bruh_decora_1_v1 (Autodesk Fusion 360 design; units mm, degrees)
Autodesk Fusion 360 part; units mm, degrees
sketch "Sketch1" plane through (0, 0, 0) normal (0, 0, 1) x (1, 0, 0)
  line L0 (0, 0) -> (125, 0)
  line L1 (125, 0) -> (125, 123.4)
  line L2 (125, 123.4) -> (0, 123.4)
  line L3 (0, 123.4) -> (0, 0)
  line L4 (24.9, 95.1) -> (54.1, 95.1)
  line L5 (56.1, 93.1) -> (56.1, 30.3)
  line L6 (54.1, 28.3) -> (24.9, 28.3)
  line L7 (22.9, 30.3) -> (22.9, 93.1)
  line L8 (22.9, 61.7) -> (57.9534, 61.7)
  line L9 (56.1, 61.7) -> (57.9534, 61.7)
  circle A0 centre (39.5, 13.3) radius 3.5
  circle A1 centre (39.5, 110.1) radius 3.5
  circle A2 centre (39.5, 110.1) radius 1.5
  circle A3 centre (39.5, 13.3) radius 1.5
  line L10 (125, 61.7) -> (0, 61.7)
  arc A4 (22.9, 30.3) -> (24.9, 28.3) centre (24.9, 30.3) ccw
  arc A5 (54.1, 28.3) -> (56.1, 30.3) centre (54.1, 30.3) ccw
  arc A6 (56.1, 93.1) -> (54.1, 95.1) centre (54.1, 93.1) ccw
  arc A7 (24.9, 95.1) -> (22.9, 93.1) centre (24.9, 93.1) ccw
  line L11 (39.5, 123.4) -> (39.5, 0)
  circle A8 centre (85.5, 110.1) radius 1.5
  circle A9 centre (85.5, 110.1) radius 3.5
  circle A10 centre (85.5, 13.3) radius 3.5
  circle A11 centre (85.5, 13.3) radius 1.5
  line L12 (70.9, 28.3) -> (100.1, 28.3)
  line L13 (102.1, 30.3) -> (102.1, 93.1)
  line L14 (100.1, 95.1) -> (70.9, 95.1)
  line L15 (68.9, 93.1) -> (68.9, 30.3)
  line L16 (85.5, 123.4) -> (85.5, 0)
  line L17 (62.5, 0) -> (62.5, 123.4)
  arc A12 (102.1, 93.1) -> (100.1, 95.1) centre (100.1, 93.1) ccw
  arc A13 (70.9, 95.1) -> (68.9, 93.1) centre (70.9, 93.1) ccw
  arc A14 (100.1, 28.3) -> (102.1, 30.3) centre (100.1, 30.3) ccw
  arc A15 (68.9, 30.3) -> (70.9, 28.3) centre (70.9, 30.3) ccw
  point P0 (56.1, 95.1)
  point P1 (56.1, 28.3)
  point P2 (22.9, 28.3)
  point P3 (39.5, 28.3)
  point P4 (39.5, 95.1)
  point P5 (68.9, 28.3)
  point P6 (102.1, 28.3)
  point P7 (102.1, 95.1)
  point P8 (68.9, 61.7)
  point P9 (102.1, 61.7)
  point P10 (85.5, 95.1)
  point P11 (85.5, 28.3)
  dimension "d1" = 123.4
  dimension "d2" = 125
  dimension "d3" = 48.4
  dimension "d4" = 48.4
  dimension "d5" = 7
  dimension "d6" = 7
  dimension "d7" = 3
  dimension "d8" = 3
  dimension "d9" = 33.2
  dimension "d10" = 66.8
  dimension "d31" = 2
  dimension "d32" = 2
  dimension "d33" = 2
  dimension "d34" = 2
  dimension "d35" = 7
  dimension "d36" = 7
  dimension "d37" = 3
  dimension "d38" = 3
  dimension "d43" = 33.2
  dimension "d44" = 66.8
  dimension "d45" = 46
  dimension "d47" = 48.4
  dimension "d48" = 48.4
  dimension "d49" = 2
  dimension "d50" = 2
  dimension "d51" = 2
  dimension "d52" = 2
  constraint horizontal L0
  constraint vertical L1
  constraint horizontal L2
  constraint vertical L3
  constraint coincident L0.start L3.end
  constraint horizontal L4
  constraint vertical L5
  constraint horizontal L6
  constraint vertical L7
  constraint perpendicular L1 L9
  constraint collinear L8 L9
  constraint concentric A1 A2
  constraint concentric A0 A3
  constraint midpoint L1 L10.start
  constraint midpoint L3 L10.end
  constraint collinear L9 L10
  constraint coincident L7 L8.start
  constraint coincident P2 L6
  constraint coincident P2 L7
  constraint tangent L6 A4
  constraint tangent L7 A4
  constraint coincident L5 L9.start
  constraint coincident P1 L5
  constraint coincident P1 L6
  constraint tangent L5 A5
  constraint tangent L6 A5
  constraint coincident P0 L4
  constraint coincident P0 L5
  constraint tangent L4 A6
  constraint tangent L5 A6
  constraint tangent L4 A7
  constraint tangent L7 A7
  constraint midpoint L7 L8.start
  constraint coincident L2 L11.start
  constraint coincident L0 L11.end
  constraint midpoint L6 P3
  constraint coincident L11 P3
  constraint midpoint L4 P4
  constraint coincident A0.centre L11
  constraint concentric A8 A9
  constraint concentric A10 A11
  constraint horizontal L12
  constraint vertical L13
  constraint horizontal L14
  constraint vertical L15
  constraint coincident L10 P8
  constraint coincident L2 L16.start
  constraint coincident L0 L16.end
  constraint perpendicular L0 L16
  constraint coincident A8.centre L16
  constraint coincident P10 L16
  constraint coincident A10.centre L16
  constraint midpoint L0 L17.start
  constraint midpoint L2 L17.end
  constraint coincident A1.centre L11
  constraint coincident L11 P4
  constraint symmetric L5 L15 L17
  constraint coincident L13 P9
  constraint coincident L14 P10
  constraint coincident P7 L13
  constraint coincident P7 L14
  constraint tangent L13 A12
  constraint tangent L14 A12
  constraint coincident L15 P8
  constraint tangent L14 A13
  constraint tangent L15 A13
  constraint coincident L12 P11
  constraint coincident P6 L12
  constraint coincident P6 L13
  constraint tangent L12 A14
  constraint tangent L13 A14
  constraint coincident P5 L12
  constraint coincident P5 L15
  constraint tangent L12 A15
  constraint tangent L15 A15
  constraint collinear L4 L14
  constraint midpoint L13 P9
  constraint midpoint L12 P11
  constraint midpoint L14 P10
  measures "d1" distance of L0.end L1.end
  measures "d2" distance of L0.start L0.end
  measures "d3" vertical distance of L8.start A0.centre
  measures "d4" vertical distance of L9.start A1.centre
  measures "d5" diameter of A0
  measures "d6" diameter of A1
  measures "d7" diameter of A2
  measures "d8" diameter of A3
  measures "d9" distance of P1 P2
  measures "d10" distance of P0 P1
  measures "d31" radius of A4
  measures "d32" radius of A5
  measures "d33" radius of A6
  measures "d34" radius of A7
  measures "d35" diameter of A10
  measures "d36" diameter of A9
  measures "d37" diameter of A8
  measures "d38" diameter of A11
  measures "d43" distance of P5 P6
  measures "d44" distance of P6 P7
  measures "d45" distance of A1.centre A8.centre
  measures "d47" vertical distance of A10.centre P8
  measures "d48" vertical distance of A8.centre P9
  measures "d49" radius of A12
  measures "d50" radius of A13
  measures "d51" radius of A14
  measures "d52" radius of A15
extrude "Extrude1" add sketch "Sketch1" along normal blind 6.4 contours L0 L3 L6 L7 A0 L10 A4 L11 | L0 L5 L6 L8 L9 A0 L10 A5 L11 L17 | L2 L3 L4 L7 A1 L10 A7 L11 | L0 L10 A10 L12 L15 L16 L17 A15 | A0 A3 L11 | A0 A3 L11 | L0 L1 L10 A10 L12 L13 L16 A14 | L2 L10 A9 L14 L15 L16 L17 A13 | L2 L4 L5 L8 L9 A1 L10 A6 L11 L17 | A10 A11 L16 | A10 A11 L16 | A1 A2 L11 | A1 A2 L11 | L1 L2 L10 A9 L13 L14 L16 A12 | A8 A9 L16 | A8 A9 L16
chamfer "Chamfer1" distance 3.5 angle 45 4 edges at (125, 61.7, 6.4) (62.5, 0, 6.4) (0, 61.7, 6.4) (62.5, 123.4, 6.4)
shell "Shell1" thickness 1.6 removed faces 1 at (7.6333, 51.2333, 0)
move_face "OffsetFaces1" offset -3.8 1 faces at (22.3667, 72.1667, 0)
move_face "OffsetFaces2" offset -4.8 1 faces at (41.8689, 109.1301, 0)
move_face "OffsetFaces3" offset -4.8 1 faces at (42.0551, 13.454, 0)
move_face "OffsetFaces4" offset -3.8 1 faces at (68.3667, 72.1667, 0)
move_face "OffsetFaces5" offset -4.8 1 faces at (83.4756, 11.7334, 0)
move_face "OffsetFaces6" offset -4.8 1 faces at (87.8689, 109.1301, 0)
chamfer "Chamfer2" distance 2 distance2 1.5 4 edges at (38.1015, 13.8424, 6.4) (84.1015, 13.8424, 6.4) (38.1015, 110.6424, 6.4) (84.1015, 110.6424, 6.4) measured on face at (9.9667, 51.2333, 6.4) measured on face at (9.9667, 51.2333, 6.4) measured on face at (9.9667, 51.2333, 6.4) measured on face at (9.9667, 51.2333, 6.4)
